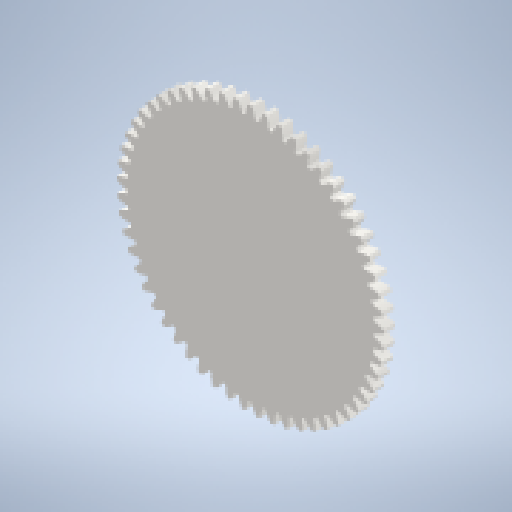
# Autodesk Inventor part: Spur Gear2
Saved by Autodesk Inventor 2023 (Build 270158000, 158)
## iProperties
Created: 2022-09-15
Part Number: Spur Gear2
Material: Steel
Document SubType Name: Modeling
Designer: simon
Categories: <?xml version="1.0" encoding="UTF-16"?> <MemberInstance><Categories><FamilyTemplate><FamilyTemplateParameter ValueType="xs:double" Id="1" ObjectReferenceKey="da_z" ObjectType="kUserParameterObject"/><FamilyTemplateParameter ValueType="xs:double" Id="2" ObjectReferenceKey="da_b" ObjectType="kUserParameterObject"/><FamilyTemplateParameter ValueType="xs:double" Id="3" ObjectReferenceKey="da_beta" ObjectType="kUserParameterObject"/><FamilyTemplateParameter ValueType="xs:double" Id="4" ObjectReferenceKey="da_da" ObjectType="kUserParameterObject"/><FamilyTemplateParameter ValueType="xs:double" Id="5" ObjectReferenceKey="da_aw" ObjectType="kUserParameterObject"/><FamilyTemplateParameter ValueType="xs:string" Id="6" ObjectReferenceKey="EAIAABAAAACIAQAAAAAAAIAAAAAAAAAA" ObjectType="83910656" SubObjectId="SurfaceGeometry"/></FamilyTemplate><ParamToTemplateMap><ParamToTemplate CategoryParameter="//CategoryParameter[@InternalName='046C89C9-8512-4d59-83FE-43B91F4F132A']" TemplateParameter="1"/><ParamToTemplate CategoryParameter="//CategoryParameter[@InternalName='2552DF32-E462-4b46-AEBF-C6C7768E72AC']" TemplateParameter="2"/><ParamToTemplate CategoryParameter="//CategoryParameter[@InternalName='C9EE641D-15FC-4fae-A226-E94C4372FDD7']" TemplateParameter="3"/><ParamToTemplate><ParamToTemplate CategoryParameter="//CategoryParameter[@InternalName='00B6519A-459B-49c7-AD84-2E56D39A5744']" ConstantValue="0.000000"/></ParamToTemplate><ParamToTemplate><ParamToTemplate CategoryParameter="//CategoryParameter[@InternalName='04B31F0E-C7A6-4894-AA32-9629BEFACF47']" ConstantValue="1.000000"/></ParamToTemplate><ParamToTemplate><ParamToTemplate CategoryParameter="//CategoryParameter[@InternalName='43CBEC2E-7847-49e7-A936-2F7889FCB2D9']" ConstantValue="0.250000"/></ParamToTemplate><ParamToTemplate><ParamToTemplate CategoryParameter="//CategoryParameter[@InternalName='B1EFC894-105D-4ebd-86BF-FA20ED196853']" ConstantValue="0.350000"/></ParamToTemplate><ParamToTemplate><ParamToTemplate CategoryParameter="//CategoryParameter[@InternalName='51175063-3D10-4879-93E8-6246FE8B403D']" ConstantValue="2060000000.000000"/></ParamToTemplate><ParamToTemplate><ParamToTemplate CategoryParameter="//CategoryParameter[@InternalName='A3A52E27-4454-46a9-B0BD-C932399B70AF']" ConstantValue="0.300000"/></ParamToTemplate><ParamToTemplate><ParamToTemplate CategoryParameter="//CategoryParameter[@InternalName='91B76062-C214-41d9-B1B9-14D2AB99603D']" ConstantValue="0.200000"/></ParamToTemplate><ParamToTemplate><ParamToTemplate CategoryParameter="//CategoryParameter[@InternalName='374E806E-8B8A-4dda-A9AA-1039D6500AD2']" ConstantValue="5.000000"/></ParamToTemplate><ParamToTemplate><ParamToTemplate CategoryParameter="//CategoryParameter[@InternalName='2D373A89-B862-43d6-8D0B-0CBF12AB9F6C']" ConstantValue="0.349066"/></ParamToTemplate><ParamToTemplate CategoryParameter="//CategoryParameter[@InternalName='37777632-D6A2-4fac-9D53-DB8ACD95C989']" TemplateParameter="4"/><ParamToTemplate CategoryParameter="//CategoryParameter[@InternalName='FD1017F1-B727-4f7e-9707-0F86F1FF9423']" TemplateParameter="5"/><ParamToTemplate><ParamToTemplate CategoryParameter="//CategoryParameter[@InternalName='9E1B4470-B2D3-4ff1-B813-535BB4CDF51A']" ConstantValue="3520000.000000"/></ParamToTemplate><ParamToTemplate><ParamToTemplate CategoryParameter="//CategoryParameter[@InternalName='F8452263-BFF6-458c-9FB1-07C4B99E95CD']" ConstantValue="11400000.000000"/></ParamToTemplate><ParamToTemplate><ParamToTemplate CategoryParameter="//CategoryParameter[@InternalName='3E3BB259-FD49-497f-8171-6EBC954A3479']" ConstantValue="2.000000"/></ParamToTemplate><ParamToTemplate CategoryParameter="//CategoryParameter[@InternalName='27C3BAF2-7550-4e4b-AE2C-0DB134B7D9B7']" TemplateParameter="6"/></ParamToTemplateMap><Category DisplayName="Gear" InternalName="DC85795E-93AB-48d5-8EEE-5A27447B64BD" Mnemonic="Gear"><CategoryParameter DisplayName="z" InternalName="046C89C9-8512-4d59-83FE-43B91F4F132A" Mnemonic="z"/><CategoryParameter DisplayName="b" InternalName="2552DF32-E462-4b46-AEBF-C6C7768E72AC" Mnemonic="b"/><CategoryParameter DisplayName="||b|" InternalName="C9EE641D-15FC-4fae-A226-E94C4372FDD7" Mnemonic="beta"/><CategoryParameter DisplayName="x" InternalName="00B6519A-459B-49c7-AD84-2E56D39A5744" Mnemonic="x"/><CategoryParameter DisplayName="a*" InternalName="04B31F0E-C7A6-4894-AA32-9629BEFACF47" Mnemonic="a"/><CategoryParameter DisplayName="c*" InternalName="43CBEC2E-7847-49e7-A936-2F7889FCB2D9" Mnemonic="c"/><CategoryParameter DisplayName="r|.f|*" InternalName="B1EFC894-105D-4ebd-86BF-FA20ED196853" Mnemonic="rf"/><CategoryParameter DisplayName="E" InternalName="51175063-3D10-4879-93E8-6246FE8B403D" Mnemonic="E"/><CategoryParameter DisplayName="||m|" InternalName="A3A52E27-4454-46a9-B0BD-C932399B70AF" Mnemonic="mi"/><Category DisplayName="SpurGear" InternalName="26C5A22E-A91E-4dfd-A3B3-23CCAFAE1764" Mnemonic="SpurGear"><CategoryParameter DisplayName="m" InternalName="91B76062-C214-41d9-B1B9-14D2AB99603D" Mnemonic="m"/><CategoryParameter DisplayName="P" InternalName="374E806E-8B8A-4dda-A9AA-1039D6500AD2" Mnemonic="PP"/><CategoryParameter DisplayName="||a|" InternalName="2D373A89-B862-43d6-8D0B-0CBF12AB9F6C" Mnemonic="alpha"/><CategoryParameter DisplayName="d|.a|" InternalName="37777632-D6A2-4fac-9D53-DB8ACD95C989" Mnemonic="da"/><CategoryParameter DisplayName="a|.w|" InternalName="FD1017F1-B727-4f7e-9707-0F86F1FF9423" Mnemonic="aw"/><CategoryParameter DisplayName="||s||.Flim|" InternalName="9E1B4470-B2D3-4ff1-B813-535BB4CDF51A" Mnemonic="sFlim"/><CategoryParameter DisplayName="||s||.Hlim|" InternalName="F8452263-BFF6-458c-9FB1-07C4B99E95CD" Mnemonic="sHlim"/><CategoryParameter DisplayName="type" InternalName="3E3BB259-FD49-497f-8171-6EBC954A3479" Mnemonic="type"/><CategoryParameter DisplayName="PitchDiameter" InternalName="27C3BAF2-7550-4e4b-AE2C-0DB134B7D9B7" Mnemonic="IDS_PITCHDIAM"/></Category></Category></Categories></MemberInstance>
Density: 1 g/cm^3
Appearance: Steel
CustomPartVersion: 1
Author: simon
Autodesk Inventor part; units mm, degrees
sketch "Sketch1" plane through (0, 0, 0) normal (0, 0, 1) x (1, 0, 0)
  circle A0 centre (0, 0) radius 59
  dimension "d0" = 118
  constraints: 1 centre point
  measures "d0" diameter of A0
extrude "Extrusion1" add sketch "Sketch1" along normal blind 5
ref_plane "Work Plane2" through (0, 0, 2.5) normal (0, 0, 1) x (1, 0, 0)
sketch "Sketch2" plane through (0, 0, 0) normal (0, 0, -1) x (-1, 0, 0)
  circle A0 centre (0, 0) radius 59 projected
  circle A1 centre (0, 0) radius 57
  dimension "d3" = 114
  constraints: 1 centre point, 1 coincident
  measures "d3" diameter of A1
surface extrude "Pitch Diameter" sketch "Sketch2" against normal through all shown no curves A1
ref_plane "Work Plane8" through (0, 0, 0) normal (0.9984815, 0.0550878, 0) x (0, 0, 1)
ref_plane "Work Plane9" through (0, 0, 0) normal (1, 0, 0) x (0, 1, 0)
spur gear teeth "Spur Gear" teeth 57 pitch diameter 114 tip diameter 118 root diameter 109 face width 20 start plane through (0, 0, 0) normal (0, 0, -1) x (-1, 0, 0)
sketch "Sketch3" plane through (0, 0, 0) normal (0, 0, -1) x (-1, 0, 0)
  arc A0 (8.2289, 53.8752) -> (7.2979, 58.5469) centre (-16.54, 51.3678) ccw projected
  arc A1 (7.2979, 58.5469) -> (5.6819, 58.7258) centre (0, 0) ccw projected
  arc A2 (5.6819, 58.7258) -> (3.7518, 54.3707) centre (27.3728, 46.5075) ccw projected
  arc A3 (3.7518, 54.3707) -> (2.2522, 54.4534) centre (0, 0) ccw projected
  arc A4 (2.2522, 54.4534) -> (0.8129, 58.9944) centre (-22.0904, 49.2365) ccw projected
  arc A5 (0.8129, 58.9944) -> (-0.8129, 58.9944) centre (0, 0) ccw projected
  arc A6 (-0.8129, 58.9944) -> (-2.2522, 54.4534) centre (22.0904, 49.2365) ccw projected
  arc A7 (-2.2522, 54.4534) -> (-3.7518, 54.3707) centre (0, 0) ccw projected
  arc A8 (-3.7518, 54.3707) -> (-5.6819, 58.7258) centre (-27.3728, 46.5075) ccw projected
  arc A9 (-5.6819, 58.7258) -> (-7.2979, 58.5469) centre (0, 0) ccw projected
  arc A10 (-7.2979, 58.5469) -> (-8.2289, 53.8752) centre (16.54, 51.3678) ccw projected
  arc A11 (-8.2289, 53.8752) -> (-9.7102, 53.628) centre (0, 0) ccw projected
  arc A12 (-9.7102, 53.628) -> (-12.1077, 57.7443) centre (-32.3229, 43.214) ccw projected
  arc A13 (-12.1077, 57.7443) -> (-13.6942, 57.3887) centre (0, 0) ccw projected
  arc A14 (-13.6942, 57.3887) -> (-14.1056, 52.643) centre (10.7887, 52.8755) ccw projected
  arc A15 (-14.1056, 52.643) -> (-15.5508, 52.2343) centre (0, 0) ccw projected
  arc A16 (-15.5508, 52.2343) -> (-18.3866, 56.0619) centre (-36.8806, 39.396) ccw projected
  arc A17 (-18.3866, 56.0619) -> (-19.9243, 55.534) centre (0, 0) ccw projected
  arc A18 (-19.9243, 55.534) -> (-19.8112, 50.7717) centre (4.9065, 53.7415) ccw projected
  arc A19 (-19.8112, 50.7717) -> (-21.2026, 50.2066) centre (0, 0) ccw projected
  arc A20 (-21.2026, 50.2066) -> (-24.4422, 53.6989) centre (-40.9906, 35.0997) ccw projected
  arc A21 (-24.4422, 53.6989) -> (-25.9126, 53.0051) centre (0, 0) ccw projected
  arc A22 (-25.9126, 53.0051) -> (-25.2762, 48.2842) centre (-1.0353, 53.955) ccw projected
  arc A23 (-25.2762, 48.2842) -> (-26.5971, 47.5694) centre (0, 0) ccw projected
  arc A24 (-26.5971, 47.5694) -> (-30.2012, 50.6842) centre (-44.6031, 30.3773) ccw projected
  arc A25 (-30.2012, 50.6842) -> (-31.5863, 49.8328) centre (0, 0) ccw projected
  arc A26 (-31.5863, 49.8328) -> (-30.4345, 45.2105) centre (-6.9645, 53.5137) ccw projected
  arc A27 (-30.4345, 45.2105) -> (-31.6687, 44.3548) centre (0, 0) ccw projected
  arc A28 (-31.6687, 44.3548) -> (-35.5936, 47.0542) centre (-47.6741, 25.2863) ccw projected
  arc A29 (-35.5936, 47.0542) -> (-36.8766, 46.0556) centre (0, 0) ccw projected
  arc A30 (-36.8766, 46.0556) -> (-35.2233, 41.5881) centre (-12.8092, 52.4227) ccw projected
  arc A31 (-35.2233, 41.5881) -> (-36.3559, 40.6017) centre (0, 0) ccw projected
  arc A32 (-36.3559, 40.6017) -> (-40.5539, 42.853) centre (-50.1665, 19.8882) ccw projected
  arc A33 (-40.5539, 42.853) -> (-41.7193, 41.7193) centre (0, 0) ccw projected
  arc A34 (-41.7193, 41.7193) -> (-39.5846, 37.4608) centre (-18.4984, 50.6954) ccw projected
  arc A35 (-39.5846, 37.4608) -> (-40.6017, 36.3559) centre (0, 0) ccw projected
  arc A36 (-40.6017, 36.3559) -> (-45.022, 38.1317) centre (-52.0499, 14.2488) ccw projected
  arc A37 (-45.022, 38.1317) -> (-46.0556, 36.8766) centre (0, 0) ccw projected
  arc A38 (-46.0556, 36.8766) -> (-43.4653, 32.8788) centre (-23.963, 48.3528) ccw projected
  arc A39 (-43.4653, 32.8788) -> (-44.3548, 31.6687) centre (0, 0) ccw projected
  arc A40 (-44.3548, 31.6687) -> (-48.9435, 32.9474) centre (-53.3015, 8.4364) ccw projected
  arc A41 (-48.9435, 32.9474) -> (-49.8328, 31.5863) centre (0, 0) ccw projected
  arc A42 (-49.8328, 31.5863) -> (-46.8184, 27.8977) centre (-29.1368, 45.4232) ccw projected
  arc A43 (-46.8184, 27.8977) -> (-47.5694, 26.5971) centre (0, 0) ccw projected
  arc A44 (-47.5694, 26.5971) -> (-52.2709, 27.3633) centre (-53.906, 2.5216) ccw projected
  arc A45 (-52.2709, 27.3633) -> (-53.0051, 25.9126) centre (0, 0) ccw projected
  arc A46 (-53.0051, 25.9126) -> (-49.6033, 22.578) centre (-33.9569, 41.9422) ccw projected
  arc A47 (-49.6033, 22.578) -> (-50.2066, 21.2026) centre (0, 0) ccw projected
  arc A48 (-50.2066, 21.2026) -> (-54.9639, 21.447) centre (-53.8563, -3.4238) ccw projected
  arc A49 (-54.9639, 21.447) -> (-55.534, 19.9243) centre (0, 0) ccw projected
  arc A50 (-55.534, 19.9243) -> (-51.786, 16.9842) centre (-38.3648, 37.9521) ccw projected
  arc A51 (-51.786, 16.9842) -> (-52.2343, 15.5508) centre (0, 0) ccw projected
  arc A52 (-52.2343, 15.5508) -> (-56.9896, 15.2703) centre (-53.1527, -9.3276) ccw projected
  arc A53 (-56.9896, 15.2703) -> (-57.3887, 13.6942) centre (0, 0) ccw projected
  arc A54 (-57.3887, 13.6942) -> (-53.3401, 11.1842) centre (-42.307, 33.5013) ccw projected
  arc A55 (-53.3401, 11.1842) -> (-53.628, 9.7102) centre (0, 0) ccw projected
  arc A56 (-53.628, 9.7102) -> (-58.3236, 8.9083) centre (-51.804, -15.1183) ccw projected
  arc A57 (-58.3236, 8.9083) -> (-58.5469, 7.2979) centre (0, 0) ccw projected
  arc A58 (-58.5469, 7.2979) -> (-54.2467, 5.2485) centre (-45.7356, 28.6439) ccw projected
  arc A59 (-54.2467, 5.2485) -> (-54.3707, 3.7518) centre (0, 0) ccw projected
  arc A60 (-54.3707, 3.7518) -> (-58.9496, 2.4382) centre (-49.8265, -20.7254) ccw projected
  arc A61 (-58.9496, 2.4382) -> (-58.9944, 0.8129) centre (0, 0) ccw projected
  arc A62 (-58.9944, 0.8129) -> (-54.4948, -0.7509) centre (-48.6091, 23.4387) ccw projected
  arc A63 (-54.4948, -0.7509) -> (-54.4534, -2.2522) centre (0, 0) ccw projected
  arc A64 (-54.4534, -2.2522) -> (-58.86, -4.0616) centre (-47.2441, -26.0809) ccw projected
  arc A65 (-58.86, -4.0616) -> (-58.7258, -5.6819) centre (0, 0) ccw projected
  arc A66 (-58.7258, -5.6819) -> (-54.0815, -6.7412) centre (-50.8925, 17.9491) ccw projected
  arc A67 (-54.0815, -6.7412) -> (-53.8752, -8.2289) centre (0, 0) ccw projected
  arc A68 (-53.8752, -8.2289) -> (-58.056, -10.512) centre (-44.0882, -31.1199) ccw projected
  arc A69 (-58.056, -10.512) -> (-57.7443, -12.1077) centre (0, 0) ccw projected
  arc A70 (-57.7443, -12.1077) -> (-53.0116, -12.6497) centre (-52.5582, 12.2415) ccw projected
  arc A71 (-53.0116, -12.6497) -> (-52.643, -14.1056) centre (0, 0) ccw projected
  arc A72 (-52.643, -14.1056) -> (-56.5472, -16.8348) centre (-40.3972, -35.7811) ccw projected
  arc A73 (-56.5472, -16.8348) -> (-56.0619, -18.3866) centre (0, 0) ccw projected
  arc A74 (-56.0619, -18.3866) -> (-51.2983, -18.4047) centre (-53.5859, 6.3854) ccw projected
  arc A75 (-51.2983, -18.4047) -> (-50.7717, -19.8112) centre (0, 0) ccw projected
  arc A76 (-50.7717, -19.8112) -> (-54.352, -22.9533) centre (-36.2158, -40.0079) ccw projected
  arc A77 (-54.352, -22.9533) -> (-53.6989, -24.4422) centre (0, 0) ccw projected
  arc A78 (-53.6989, -24.4422) -> (-48.9623, -23.9362) centre (-53.9631, 0.4518) ccw projected
  arc A79 (-48.9623, -23.9362) -> (-48.2842, -25.2762) centre (0, 0) ccw projected
  arc A80 (-48.2842, -25.2762) -> (-51.4971, -28.7932) centre (-31.5948, -43.7491) ccw projected
  arc A81 (-51.4971, -28.7932) -> (-50.6842, -30.2012) centre (0, 0) ccw projected
  arc A82 (-50.6842, -30.2012) -> (-46.032, -29.1772) centre (-53.6853, -5.4873) ccw projected
  arc A83 (-46.032, -29.1772) -> (-45.2105, -30.4345) centre (0, 0) ccw projected
  arc A84 (-45.2105, -30.4345) -> (-48.0171, -34.2835) centre (-26.5903, -46.9593) ccw projected
  arc A85 (-48.0171, -34.2835) -> (-47.0542, -35.5936) centre (0, 0) ccw projected
  arc A86 (-47.0542, -35.5936) -> (-42.5428, -34.064) centre (-52.7558, -11.3599) ccw projected
  arc A87 (-42.5428, -34.064) -> (-41.5881, -35.2233) centre (0, 0) ccw projected
  arc A88 (-41.5881, -35.2233) -> (-43.9542, -39.3577) centre (-21.263, -49.5994) ccw projected
  arc A89 (-43.9542, -39.3577) -> (-42.853, -40.5539) centre (0, 0) ccw projected
  arc A90 (-42.853, -40.5539) -> (-38.5373, -38.5373) centre (-51.1859, -17.0945) ccw projected
  arc A91 (-38.5373, -38.5373) -> (-37.4608, -39.5846) centre (0, 0) ccw projected
  arc A92 (-37.4608, -39.5846) -> (-39.3577, -43.9542) centre (-15.6776, -51.6375) ccw projected
  arc A93 (-39.3577, -43.9542) -> (-38.1317, -45.022) centre (0, 0) ccw projected
  arc A94 (-38.1317, -45.022) -> (-34.064, -42.5428) centre (-48.9947, -22.6216) ccw projected
  arc A95 (-34.064, -42.5428) -> (-32.8788, -43.4653) centre (0, 0) ccw projected
  arc A96 (-32.8788, -43.4653) -> (-34.2835, -48.0171) centre (-9.9019, -53.0488) ccw projected
  arc A97 (-34.2835, -48.0171) -> (-32.9474, -48.9435) centre (0, 0) ccw projected
  arc A98 (-32.9474, -48.9435) -> (-29.1772, -46.032) centre (-46.2088, -27.8741) ccw projected
  arc A99 (-29.1772, -46.032) -> (-27.8977, -46.8184) centre (0, 0) ccw projected
  arc A100 (-27.8977, -46.8184) -> (-28.7932, -51.4971) centre (-4.006, -53.8161) ccw projected
  arc A101 (-28.7932, -51.4971) -> (-27.3633, -52.2709) centre (0, 0) ccw projected
  arc A102 (-27.3633, -52.2709) -> (-23.9362, -48.9623) centre (-42.8619, -32.7883) ccw projected
  arc A103 (-23.9362, -48.9623) -> (-22.578, -49.6033) centre (0, 0) ccw projected
  arc A104 (-22.578, -49.6033) -> (-22.9533, -54.352) centre (1.9385, -53.9301) ccw projected
  arc A105 (-22.9533, -54.352) -> (-21.447, -54.9639) centre (0, 0) ccw projected
  arc A106 (-21.447, -54.9639) -> (-18.4047, -51.2983) centre (-38.9948, -37.3045) ccw projected
  arc A107 (-18.4047, -51.2983) -> (-16.9842, -51.786) centre (0, 0) ccw projected
  arc A108 (-16.9842, -51.786) -> (-16.8348, -56.5472) centre (7.8595, -53.3896) ccw projected
  arc A109 (-16.8348, -56.5472) -> (-15.2703, -56.9896) centre (0, 0) ccw projected
  arc A110 (-15.2703, -56.9896) -> (-12.6497, -53.0116) centre (-34.6543, -41.3678) ccw projected
  arc A111 (-12.6497, -53.0116) -> (-11.1842, -53.3401) centre (0, 0) ccw projected
  arc A112 (-11.1842, -53.3401) -> (-10.512, -58.056) centre (13.6851, -52.2009) ccw projected
  arc A113 (-10.512, -58.056) -> (-8.9083, -58.3236) centre (0, 0) ccw projected
  arc A114 (-8.9083, -58.3236) -> (-6.7412, -54.0815) centre (-29.8932, -44.929) ccw projected
  arc A115 (-6.7412, -54.0815) -> (-5.2485, -54.2467) centre (0, 0) ccw projected
  arc A116 (-5.2485, -54.2467) -> (-4.0616, -58.86) centre (19.3446, -50.3786) ccw projected
  arc A117 (-4.0616, -58.86) -> (-2.4382, -58.9496) centre (0, 0) ccw projected
  arc A118 (-2.4382, -58.9496) -> (-0.7509, -54.4948) centre (-24.7692, -47.9448) ccw projected
  arc A119 (-0.7509, -54.4948) -> (0.7509, -54.4948) centre (0, 0) ccw projected
  arc A120 (0.7509, -54.4948) -> (2.4382, -58.9496) centre (24.7692, -47.9448) ccw projected
  arc A121 (2.4382, -58.9496) -> (4.0616, -58.86) centre (0, 0) ccw projected
  arc A122 (4.0616, -58.86) -> (5.2485, -54.2467) centre (-19.3446, -50.3786) ccw projected
  arc A123 (5.2485, -54.2467) -> (6.7412, -54.0815) centre (0, 0) ccw projected
  arc A124 (6.7412, -54.0815) -> (8.9083, -58.3236) centre (29.8932, -44.929) ccw projected
  arc A125 (8.9083, -58.3236) -> (10.512, -58.056) centre (0, 0) ccw projected
  arc A126 (10.512, -58.056) -> (11.1842, -53.3401) centre (-13.6851, -52.2009) ccw projected
  arc A127 (11.1842, -53.3401) -> (12.6497, -53.0116) centre (0, 0) ccw projected
  arc A128 (12.6497, -53.0116) -> (15.2703, -56.9896) centre (34.6543, -41.3678) ccw projected
  arc A129 (15.2703, -56.9896) -> (16.8348, -56.5472) centre (0, 0) ccw projected
  arc A130 (16.8348, -56.5472) -> (16.9842, -51.786) centre (-7.8595, -53.3896) ccw projected
  arc A131 (16.9842, -51.786) -> (18.4047, -51.2983) centre (0, 0) ccw projected
  arc A132 (18.4047, -51.2983) -> (21.447, -54.9639) centre (38.9948, -37.3045) ccw projected
  arc A133 (21.447, -54.9639) -> (22.9533, -54.352) centre (0, 0) ccw projected
  arc A134 (22.9533, -54.352) -> (22.578, -49.6033) centre (-1.9385, -53.9301) ccw projected
  arc A135 (22.578, -49.6033) -> (23.9362, -48.9623) centre (0, 0) ccw projected
  arc A136 (23.9362, -48.9623) -> (27.3633, -52.2709) centre (42.8619, -32.7883) ccw projected
  arc A137 (27.3633, -52.2709) -> (28.7932, -51.4971) centre (0, 0) ccw projected
  arc A138 (28.7932, -51.4971) -> (27.8977, -46.8184) centre (4.006, -53.8161) ccw projected
  arc A139 (27.8977, -46.8184) -> (29.1772, -46.032) centre (0, 0) ccw projected
  arc A140 (29.1772, -46.032) -> (32.9474, -48.9435) centre (46.2088, -27.8741) ccw projected
  arc A141 (32.9474, -48.9435) -> (34.2835, -48.0171) centre (0, 0) ccw projected
  arc A142 (34.2835, -48.0171) -> (32.8788, -43.4653) centre (9.9019, -53.0488) ccw projected
  arc A143 (32.8788, -43.4653) -> (34.064, -42.5428) centre (0, 0) ccw projected
  arc A144 (34.064, -42.5428) -> (38.1317, -45.022) centre (48.9947, -22.6216) ccw projected
  arc A145 (38.1317, -45.022) -> (39.3577, -43.9542) centre (0, 0) ccw projected
  arc A146 (39.3577, -43.9542) -> (37.4608, -39.5846) centre (15.6776, -51.6375) ccw projected
  arc A147 (37.4608, -39.5846) -> (38.5373, -38.5373) centre (0, 0) ccw projected
  arc A148 (38.5373, -38.5373) -> (42.853, -40.5539) centre (51.1859, -17.0945) ccw projected
  arc A149 (42.853, -40.5539) -> (43.9542, -39.3577) centre (0, 0) ccw projected
  arc A150 (43.9542, -39.3577) -> (41.5881, -35.2233) centre (21.263, -49.5994) ccw projected
  arc A151 (41.5881, -35.2233) -> (42.5428, -34.064) centre (0, 0) ccw projected
  arc A152 (42.5428, -34.064) -> (47.0542, -35.5936) centre (52.7558, -11.3599) ccw projected
  arc A153 (47.0542, -35.5936) -> (48.0171, -34.2835) centre (0, 0) ccw projected
  arc A154 (48.0171, -34.2835) -> (45.2105, -30.4345) centre (26.5903, -46.9593) ccw projected
  arc A155 (45.2105, -30.4345) -> (46.032, -29.1772) centre (0, 0) ccw projected
  arc A156 (46.032, -29.1772) -> (50.6842, -30.2012) centre (53.6853, -5.4873) ccw projected
  arc A157 (50.6842, -30.2012) -> (51.4971, -28.7932) centre (0, 0) ccw projected
  arc A158 (51.4971, -28.7932) -> (48.2842, -25.2762) centre (31.5948, -43.7491) ccw projected
  arc A159 (48.2842, -25.2762) -> (48.9623, -23.9362) centre (0, 0) ccw projected
  arc A160 (48.9623, -23.9362) -> (53.6989, -24.4422) centre (53.9631, 0.4518) ccw projected
  arc A161 (53.6989, -24.4422) -> (54.352, -22.9533) centre (0, 0) ccw projected
  arc A162 (54.352, -22.9533) -> (50.7717, -19.8112) centre (36.2158, -40.0079) ccw projected
  arc A163 (50.7717, -19.8112) -> (51.2983, -18.4047) centre (0, 0) ccw projected
  arc A164 (51.2983, -18.4047) -> (56.0619, -18.3866) centre (53.5859, 6.3854) ccw projected
  arc A165 (56.0619, -18.3866) -> (56.5472, -16.8348) centre (0, 0) ccw projected
  arc A166 (56.5472, -16.8348) -> (52.643, -14.1056) centre (40.3972, -35.7811) ccw projected
  arc A167 (52.643, -14.1056) -> (53.0116, -12.6497) centre (0, 0) ccw projected
  arc A168 (53.0116, -12.6497) -> (57.7443, -12.1077) centre (52.5582, 12.2415) ccw projected
  arc A169 (57.7443, -12.1077) -> (58.056, -10.512) centre (0, 0) ccw projected
  arc A170 (58.056, -10.512) -> (53.8752, -8.2289) centre (44.0882, -31.1199) ccw projected
  arc A171 (53.8752, -8.2289) -> (54.0815, -6.7412) centre (0, 0) ccw projected
  arc A172 (54.0815, -6.7412) -> (58.7258, -5.6819) centre (50.8925, 17.9491) ccw projected
  arc A173 (58.7258, -5.6819) -> (58.86, -4.0616) centre (0, 0) ccw projected
  arc A174 (58.86, -4.0616) -> (54.4534, -2.2522) centre (47.2441, -26.0809) ccw projected
  arc A175 (54.4534, -2.2522) -> (54.4948, -0.7509) centre (0, 0) ccw projected
  arc A176 (54.4948, -0.7509) -> (58.9944, 0.8129) centre (48.6091, 23.4387) ccw projected
  arc A177 (58.9944, 0.8129) -> (58.9496, 2.4382) centre (0, 0) ccw projected
  arc A178 (58.9496, 2.4382) -> (54.3707, 3.7518) centre (49.8265, -20.7254) ccw projected
  arc A179 (54.3707, 3.7518) -> (54.2467, 5.2485) centre (0, 0) ccw projected
  arc A180 (54.2467, 5.2485) -> (58.5469, 7.2979) centre (45.7356, 28.6439) ccw projected
  arc A181 (58.5469, 7.2979) -> (58.3236, 8.9083) centre (0, 0) ccw projected
  arc A182 (58.3236, 8.9083) -> (53.628, 9.7102) centre (51.804, -15.1183) ccw projected
  arc A183 (53.628, 9.7102) -> (53.3401, 11.1842) centre (0, 0) ccw projected
  arc A184 (53.3401, 11.1842) -> (57.3887, 13.6942) centre (42.307, 33.5013) ccw projected
  arc A185 (57.3887, 13.6942) -> (56.9896, 15.2703) centre (0, 0) ccw projected
  arc A186 (56.9896, 15.2703) -> (52.2343, 15.5508) centre (53.1527, -9.3276) ccw projected
  arc A187 (52.2343, 15.5508) -> (51.786, 16.9842) centre (0, 0) ccw projected
  arc A188 (51.786, 16.9842) -> (55.534, 19.9243) centre (38.3648, 37.9521) ccw projected
  arc A189 (55.534, 19.9243) -> (54.9639, 21.447) centre (0, 0) ccw projected
  arc A190 (54.9639, 21.447) -> (50.2066, 21.2026) centre (53.8563, -3.4238) ccw projected
  arc A191 (50.2066, 21.2026) -> (49.6033, 22.578) centre (0, 0) ccw projected
  arc A192 (49.6033, 22.578) -> (53.0051, 25.9126) centre (33.9569, 41.9422) ccw projected
  arc A193 (53.0051, 25.9126) -> (52.2709, 27.3633) centre (0, 0) ccw projected
  arc A194 (52.2709, 27.3633) -> (47.5694, 26.5971) centre (53.906, 2.5216) ccw projected
  arc A195 (47.5694, 26.5971) -> (46.8184, 27.8977) centre (0, 0) ccw projected
  arc A196 (46.8184, 27.8977) -> (49.8328, 31.5863) centre (29.1368, 45.4232) ccw projected
  arc A197 (49.8328, 31.5863) -> (48.9435, 32.9474) centre (0, 0) ccw projected
  arc A198 (48.9435, 32.9474) -> (44.3548, 31.6687) centre (53.3015, 8.4364) ccw projected
  arc A199 (44.3548, 31.6687) -> (43.4653, 32.8788) centre (0, 0) ccw projected
  arc A200 (43.4653, 32.8788) -> (46.0556, 36.8766) centre (23.963, 48.3528) ccw projected
  arc A201 (46.0556, 36.8766) -> (45.022, 38.1317) centre (0, 0) ccw projected
  arc A202 (45.022, 38.1317) -> (40.6017, 36.3559) centre (52.0499, 14.2488) ccw projected
  arc A203 (40.6017, 36.3559) -> (39.5846, 37.4608) centre (0, 0) ccw projected
  arc A204 (39.5846, 37.4608) -> (41.7193, 41.7193) centre (18.4984, 50.6954) ccw projected
  arc A205 (41.7193, 41.7193) -> (40.5539, 42.853) centre (0, 0) ccw projected
  arc A206 (40.5539, 42.853) -> (36.3559, 40.6017) centre (50.1665, 19.8882) ccw projected
  arc A207 (36.3559, 40.6017) -> (35.2233, 41.5881) centre (0, 0) ccw projected
  arc A208 (35.2233, 41.5881) -> (36.8766, 46.0556) centre (12.8092, 52.4227) ccw projected
  arc A209 (36.8766, 46.0556) -> (35.5936, 47.0542) centre (0, 0) ccw projected
  arc A210 (35.5936, 47.0542) -> (31.6687, 44.3548) centre (47.6741, 25.2863) ccw projected
  arc A211 (31.6687, 44.3548) -> (30.4345, 45.2105) centre (0, 0) ccw projected
  arc A212 (30.4345, 45.2105) -> (31.5863, 49.8328) centre (6.9645, 53.5137) ccw projected
  arc A213 (31.5863, 49.8328) -> (30.2012, 50.6842) centre (0, 0) ccw projected
  arc A214 (30.2012, 50.6842) -> (26.5971, 47.5694) centre (44.6031, 30.3773) ccw projected
  arc A215 (26.5971, 47.5694) -> (25.2762, 48.2842) centre (0, 0) ccw projected
  arc A216 (25.2762, 48.2842) -> (25.9126, 53.0051) centre (1.0353, 53.955) ccw projected
  arc A217 (25.9126, 53.0051) -> (24.4422, 53.6989) centre (0, 0) ccw projected
  arc A218 (24.4422, 53.6989) -> (21.2026, 50.2066) centre (40.9906, 35.0997) ccw projected
  arc A219 (21.2026, 50.2066) -> (19.8112, 50.7717) centre (0, 0) ccw projected
  arc A220 (19.8112, 50.7717) -> (19.9243, 55.534) centre (-4.9065, 53.7415) ccw projected
  arc A221 (19.9243, 55.534) -> (18.3866, 56.0619) centre (0, 0) ccw projected
  arc A222 (18.3866, 56.0619) -> (15.5508, 52.2343) centre (36.8806, 39.396) ccw projected
  arc A223 (15.5508, 52.2343) -> (14.1056, 52.643) centre (0, 0) ccw projected
  arc A224 (14.1056, 52.643) -> (13.6942, 57.3887) centre (-10.7887, 52.8755) ccw projected
  arc A225 (13.6942, 57.3887) -> (12.1077, 57.7443) centre (0, 0) ccw projected
  arc A226 (12.1077, 57.7443) -> (9.7102, 53.628) centre (32.3229, 43.214) ccw projected
  arc A227 (9.7102, 53.628) -> (8.2289, 53.8752) centre (0, 0) ccw projected
  circle A228 centre (0, 0) radius 4.9
  dimension "d49" = 9.8
  constraints: 1 centre point, 1 coincident
  measures "d49" diameter of A228
extrude "Extrusion2" add sketch "Sketch3" along normal blind 36 contours A228
equation "\"d0\" = da_da"
equation "\"d3\" = da_d"
equation "\"da_da\" = 118"
equation "\"da_d\" = 114"
body "Solid1"
body "Srf1"
